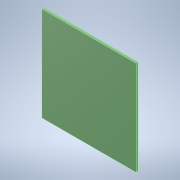
# Autodesk Inventor part: PCB-Bottom
Saved by Autodesk Inventor 2022 (Build 260153000, 153)
## iProperties
Created: 2024-05-30
Part Number: PCB-Bottom
Material: 一般
Document SubType Name: Modeling
Designer: yamashita1
Density: 1 g/cm^3
Appearance: 滑らか - 濃い深緑
Author: yamashita1
Autodesk Inventor part; units mm, degrees
ref_plane "YZ Plane" through (0, 0, 0) normal (1, 0, 0) x (0, 1, 0)
ref_plane "XZ Plane" through (0, 0, 0) normal (0, 1, 0) x (-1, 0, 0)
ref_plane "XY Plane" through (0, 0, 0) normal (0, 0, 1) x (1, 0, 0)
sketch "スケッチ1" plane through (0, 0, 0) normal (0, 0, 1) x (1, 0, 0)
  line L0 (-35, 35) -> (35, 35)
  line L1 (35, 35) -> (35, -35)
  line L2 (35, -35) -> (-35, -35)
  line L3 (-35, -35) -> (-35, 35)
  point P0 (0, 0)
  point P1 (0, 35)
  point P2 (-35, 0)
  dimension "d0" = 70
  dimension "d1" = 70
  constraints: 8 end point, 2 midpoint, 2 parallel, 1 horizontal, 1 horizontal alignment, 1 perpendicular, 1 vertical alignment
  measures "d0" distance of L1.end L2.end
  measures "d1" distance of L0.end L1.end
extrude "押し出し1" add sketch "スケッチ1" along normal blind 1.6
